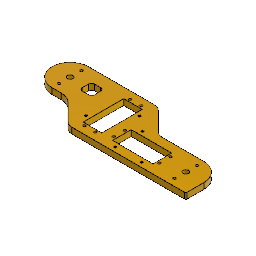
grt_thigh_20190218 (Autodesk Fusion 360 design; units mm, degrees)
Autodesk Fusion 360 part; units mm, degrees
note: some values were not read from the file. Set by a fixed rule: which sketch regions a step uses.
sketch "Sketch" plane through (0, 0, 0) normal (0, 1, 0) x (-1, 0, 0)
  circle A0 centre (115, -20) radius 4.5
  circle A1 centre (-115, 20) radius 4.5
  circle A2 centre (115, -38.5) radius 2.1
  circle A3 centre (115, -1.5) radius 2.1
  line L0 (115, 10) -> (99.5972, 10)
  line L1 (81.0587, 17.6789) -> (53.131, 45.6066)
  line L2 (42.5244, 50) -> (-143, 50)
  line L3 (115, -50) -> (20.0095, -50)
  arc A4 (81.0587, 17.6789) -> (99.5972, 10) centre (99.5972, 36.2173) ccw
  arc A5 (53.131, 45.6066) -> (42.5244, 50) centre (42.5244, 35) ccw
  circle A6 centre (-115, 38.5) radius 2.1
  circle A7 centre (-115, 1.5) radius 2.1
  line L4 (-116.33, -10) -> (-46.2132, -10)
  line L5 (-145, 48) -> (-145, 19.9705)
  arc A8 (-145, 19.9705) -> (-116.33, -10) centre (-115, 19.9705) ccw
  line L6 (6.2132, -50) -> (20.0095, -50)
  line L7 (-35.6066, -14.3934) -> (-4.3934, -45.6066)
  arc A9 (115, -50) -> (115, 10) centre (115, -20) ccw
  line L8 (40.268, -33.25) -> (40.268, 33.25)
  line L9 (9.768, -33.25) -> (40.268, -33.25)
  line L10 (40.268, 33.25) -> (9.768, 33.25)
  line L11 (9.768, 33.25) -> (9.768, -33.25)
  circle A10 centre (16.018, 37.5) radius 2.05
  circle A11 centre (16.018, -37.5) radius 2.05
  circle A12 centre (34.018, -37.5) radius 2.05
  circle A13 centre (34.018, 37.5) radius 2.05
  line L12 (-76.45, 4.75) -> (-9.95, 4.75)
  line L13 (-76.45, 35.25) -> (-76.45, 4.75)
  line L14 (-9.95, 4.75) -> (-9.95, 35.25)
  line L15 (-9.95, 35.25) -> (-76.45, 35.25)
  circle A14 centre (-5.7, 29) radius 2.05
  circle A15 centre (-80.7, 29) radius 2.05
  circle A16 centre (-80.7, 11) radius 2.05
  circle A17 centre (-5.7, 11) radius 2.05
  arc A18 (-4.3934, -45.6066) -> (6.2132, -50) centre (6.2132, -35) ccw
  arc A19 (-35.6066, -14.3934) -> (-46.2132, -10) centre (-46.2132, -25) ccw
  line L16 (85, -30) -> (75, -30)
  line L17 (70, -25) -> (70, -15)
  line L18 (75, -10) -> (85, -10)
  line L19 (90, -15) -> (90, -25)
  arc A20 (85, -30) -> (90, -25) centre (85, -25) ccw
  arc A21 (90, -15) -> (85, -10) centre (85, -15) ccw
  arc A22 (75, -10) -> (70, -15) centre (75, -15) ccw
  arc A23 (70, -25) -> (75, -30) centre (75, -25) ccw
  arc A24 (-143, 50) -> (-145, 48) centre (-143, 48) ccw
  dimension "d1" = 9
  dimension "d15" = 4.2
  dimension "d16" = 18.5
  dimension "d17" = 37
  dimension "d24" = 135
  dimension "d25" = 60
  dimension "d36" = 30
  dimension "d40" = 15
  dimension "d86" = 4.2
  dimension "d87" = 4.2
  dimension "d88" = 37
  dimension "d89" = 18.5
  dimension "d98" = 100
  dimension "d99" = 115
  dimension "d100" = 50
  dimension "d105" = 30
  dimension "d109" = 75
  dimension "d110" = 230
  dimension "d111" = 30
  dimension "d112" = 30
  dimension "d157" = 15.25
  dimension "d158" = 15.25
  dimension "d159" = 33.25
  dimension "d160" = 33.25
  dimension "d161" = 4.1
  dimension "d162" = 18
  dimension "d163" = 75
  dimension "d167" = 15.25
  dimension "d168" = 9
  dimension "d169" = 37.5
  dimension "d170" = 18
  dimension "d172" = 15.25
  dimension "d173" = 15.25
  dimension "d174" = 33.25
  dimension "d175" = 33.25
  dimension "d176" = 4.1
  dimension "d177" = 18
  dimension "d178" = 75
  dimension "d181" = 18.2
  dimension "d182" = 15.25
  dimension "d183" = 37.5
  dimension "d184" = 9
  dimension "d185" = 90
  dimension "d228" = 15
  dimension "d229" = 15
  dimension "d230" = 5
  dimension "d231" = 20
  dimension "d232" = 25
  dimension "d233" = 135
  dimension "d234" = 2
  dimension "d270" = 18.2
  dimension "d271" = 90
  measures "d1" diameter of A0
  measures "d15" diameter of A2
  measures "d16" distance of origin
  measures "d17" distance of origin
  measures "d24" angle of L0 L1
  measures "d25" distance of origin
  measures "d40" radius of A5
  measures "d86" diameter of A6
  measures "d87" diameter of A7
  measures "d88" distance of origin
  measures "d98" distance of L2 L3
  measures "d99" distance of origin
  measures "d109" distance of origin
  measures "d111" distance of origin L4
  measures "d112" distance of origin L5
  measures "d158" distance of origin L11
  measures "d159" distance of origin L10
  measures "d160" distance of origin L9
  measures "d161" diameter of A13
  measures "d162" distance of origin
  measures "d168" distance of origin
  measures "d170" distance of origin
  measures "d172" distance of L12
  measures "d173" distance of L15
  measures "d174" distance of L14
  measures "d175" distance of L13
  measures "d176" diameter of A17
  measures "d182" distance of L12
  measures "d185" distance of origin
  measures "d228" radius of A18
  measures "d229" radius of A19
  measures "d230" radius of A20
  measures "d231" distance of L3 L16
  measures "d232" distance of L19
  measures "d233" angle of L4 L7
  measures "d234" radius of A24
  measures "d270" distance of origin
extrude "Extrusion2" add sketch "Sketch" along normal blind 10
sketch "Skizze3" plane through (0, 10, 0) normal (0, 1, 0) x (-1, 0, 0)
  circle A0 centre (16.018, 37.5) radius 2.05
  circle A1 centre (16.018, -37.5) radius 2.05
  circle A2 centre (34.018, -37.5) radius 2.05
  circle A3 centre (34.018, 37.5) radius 2.05
  circle A4 centre (-115, 1.5) radius 2.1
  line L0 (9.768, -33.25) -> (9.768, 33.25)
  line L1 (9.768, 33.25) -> (40.268, 33.25)
  line L2 (40.268, 33.25) -> (40.268, -33.25)
  line L3 (40.268, -33.25) -> (9.768, -33.25)
  circle A5 centre (-115, 38.5) radius 2.1
  circle A6 centre (115, -1.5) radius 2.1
  circle A7 centre (115, -38.5) radius 2.1
  circle A8 centre (-115, 20) radius 4.5
  circle A9 centre (115, -20) radius 4.5
  circle A10 centre (-80.7, 11) radius 2.05
  circle A11 centre (-5.7, 11) radius 2.05
  circle A12 centre (-80.7, 29) radius 2.05
  circle A13 centre (-5.7, 29) radius 2.05
  line L4 (-76.45, 35.25) -> (-9.95, 35.25)
  line L5 (-9.95, 35.25) -> (-9.95, 4.75)
  line L6 (-9.95, 4.75) -> (-76.45, 4.75)
  line L7 (-76.45, 4.75) -> (-76.45, 35.25)
  line L8 (81.0587, 17.6789) -> (53.131, 45.6066)
  arc A14 (53.131, 45.6066) -> (42.5244, 50) centre (42.5244, 35) ccw
  line L9 (42.5244, 50) -> (-143, 50)
  line L10 (-145, 48) -> (-145, 19.9705)
  arc A15 (-145, 19.9705) -> (-116.33, -10) centre (-115, 19.9705) ccw
  line L11 (-116.33, -10) -> (-46.2132, -10)
  line L12 (-35.6066, -14.3934) -> (-4.3934, -45.6066)
  line L13 (6.2132, -50) -> (115, -50)
  arc A16 (115, -50) -> (115, 10) centre (115, -20) ccw
  line L14 (115, 10) -> (99.5972, 10)
  arc A17 (81.0587, 17.6789) -> (99.5972, 10) centre (99.5972, 36.2173) ccw
  line L15 (6.2132, -50) -> (20.0095, -50)
  line L16 (115, -50) -> (20.0095, -50)
  line L17 (42.5244, 50) -> (-143, 50)
  arc A18 (-4.3934, -45.6066) -> (6.2132, -50) centre (6.2132, -35) ccw
  arc A19 (-35.6066, -14.3934) -> (-46.2132, -10) centre (-46.2132, -25) ccw
  arc A20 (75, -10) -> (70, -15) centre (75, -15) ccw
  line L18 (75, -10) -> (85, -10)
  arc A21 (90, -15) -> (85, -10) centre (85, -15) ccw
  line L19 (90, -15) -> (90, -25)
  arc A22 (85, -30) -> (90, -25) centre (85, -25) ccw
  line L20 (85, -30) -> (75, -30)
  arc A23 (70, -25) -> (75, -30) centre (75, -25) ccw
  line L21 (70, -25) -> (70, -15)
  arc A24 (-143, 50) -> (-145, 48) centre (-143, 48) ccw
  line L22 (48.268, 20.25) -> (46.268, 20.25)
  line L23 (45.768, 20.75) -> (45.768, 22.75)
  line L24 (46.268, 23.25) -> (48.268, 23.25)
  line L25 (48.768, 22.75) -> (48.768, 20.75)
  arc A25 (48.768, 22.75) -> (48.268, 23.25) centre (48.268, 22.75) ccw
  arc A26 (48.268, 20.25) -> (48.768, 20.75) centre (48.268, 20.75) ccw
  arc A27 (45.768, 20.75) -> (46.268, 20.25) centre (46.268, 20.75) ccw
  arc A28 (46.268, 23.25) -> (45.768, 22.75) centre (46.268, 22.75) ccw
  line L26 (1.268, -22.75) -> (1.268, -20.75)
  arc A29 (3.768, -23.25) -> (4.268, -22.75) centre (3.768, -22.75) ccw
  arc A30 (1.768, -20.25) -> (1.268, -20.75) centre (1.768, -20.75) ccw
  line L27 (1.768, -20.25) -> (3.768, -20.25)
  arc A31 (4.268, -20.75) -> (3.768, -20.25) centre (3.768, -20.75) ccw
  line L28 (4.268, -20.75) -> (4.268, -22.75)
  arc A32 (1.268, -22.75) -> (1.768, -23.25) centre (1.768, -22.75) ccw
  line L29 (3.768, -23.25) -> (1.768, -23.25)
  line L30 (-22.95, 41.5) -> (-22.95, 43.5)
  arc A33 (-20.45, 41) -> (-19.95, 41.5) centre (-20.45, 41.5) ccw
  arc A34 (-22.45, 44) -> (-22.95, 43.5) centre (-22.45, 43.5) ccw
  line L31 (-22.45, 44) -> (-20.45, 44)
  arc A35 (-19.95, 43.5) -> (-20.45, 44) centre (-20.45, 43.5) ccw
  line L32 (-19.95, 43.5) -> (-19.95, 41.5)
  arc A36 (-22.95, 41.5) -> (-22.45, 41) centre (-22.45, 41.5) ccw
  line L33 (-20.45, 41) -> (-22.45, 41)
  line L34 (-66.45, 41.5) -> (-66.45, 43.5)
  arc A37 (-63.95, 41) -> (-63.45, 41.5) centre (-63.95, 41.5) ccw
  arc A38 (-65.95, 44) -> (-66.45, 43.5) centre (-65.95, 43.5) ccw
  line L35 (-65.95, 44) -> (-63.95, 44)
  arc A39 (-63.45, 43.5) -> (-63.95, 44) centre (-63.95, 43.5) ccw
  line L36 (-63.45, 43.5) -> (-63.45, 41.5)
  arc A40 (-66.45, 41.5) -> (-65.95, 41) centre (-65.95, 41.5) ccw
  line L37 (-63.95, 41) -> (-65.95, 41)
  line L38 (-20.45, -3.75) -> (-22.45, -3.75)
  line L39 (-19.95, -1.25) -> (-19.95, -3.25)
  arc A41 (-20.45, -3.75) -> (-19.95, -3.25) centre (-20.45, -3.25) ccw
  arc A42 (-22.45, -0.75) -> (-22.95, -1.25) centre (-22.45, -1.25) ccw
  arc A43 (-22.95, -3.25) -> (-22.45, -3.75) centre (-22.45, -3.25) ccw
  line L40 (-22.95, -3.25) -> (-22.95, -1.25)
  line L41 (-22.45, -0.75) -> (-20.45, -0.75)
  arc A44 (-19.95, -1.25) -> (-20.45, -0.75) centre (-20.45, -1.25) ccw
  point P0 (-269.883, 0)
  dimension "d235" = 3
  dimension "d236" = 3
  dimension "d237" = 0.5
  dimension "d238" = 10
  dimension "d239" = 5.5
  dimension "d240" = 3
  dimension "d241" = 3
  dimension "d242" = 0.5
  dimension "d244" = 5.5
  dimension "d245" = 3
  dimension "d246" = 3
  dimension "d247" = 0.5
  dimension "d248" = 6
  dimension "d251" = 10
  dimension "d255" = 3
  dimension "d256" = 3
  dimension "d257" = 0.5
  dimension "d260" = 10
  dimension "d261" = 6
  dimension "d262" = 10
  dimension "d263" = 3
  dimension "d264" = 3
  dimension "d265" = 0.5
  dimension "d266" = 10
  dimension "d267" = 5.5
  measures "d237" radius of A25
  measures "d238" distance of L1 L24
  measures "d239" distance of L2 L23
  measures "d240" distance of P0
  measures "d242" radius of A31
  measures "d244" distance of L0 L28
  measures "d245" distance of origin
  measures "d247" radius of A35
  measures "d248" distance of L9 L31
  measures "d251" distance of L5 L32
  measures "d257" radius of A39
  measures "d260" distance of L7 L34
  measures "d261" distance of L9 L35
  measures "d262" distance of L3 L29
  measures "d265" radius of A44
  measures "d266" distance of L5 L39
  measures "d267" distance of L6 L41
extrude "Extrusion5" cut sketch "Skizze3" against normal blind 10 contours L22 L23 L24 L25 A25 A26 A27 A28 | L26 A29 A30 L27 A31 L28 A32 L29 | L30 A33 A34 L31 A35 L32 A36 L33 | L34 A37 A38 L35 A39 L36 A40 L37 | L38 L39 A41 A42 A43 L40 L41 A44
equation "Belt_Diameter = 90 mm"
equation "d157 = 15 mm + tolerance"
equation "d158 = 15 mm + tolerance"
equation "d159 = 33 mm + tolerance"
equation "d160 = 33 mm + tolerance"
equation "d167 = 15 mm + tolerance"
equation "d172 = 15 mm + tolerance"
equation "d173 = 15 mm + tolerance"
equation "d174 = 33 mm + tolerance"
equation "d175 = 33 mm + tolerance"
equation "d182 = 15 mm + tolerance"
equation "tolerance = 0.25 mm"
